Autodesk Inventor part; units mm, degrees
(part 2 of 3)
sketch "Sketch6" plane through (-41.727, 100.5291, 48.8096) normal (0.258819, 0.9659258, 0) x (0.9659258, -0.258819, 0)
  line L0 (0, 0) -> (0, 97.6191) projected
  line L1 (17.5553, 17.379) -> (17.5553, 16.4322)
  line L2 (17.5553, 16.4322) -> (12.0801, 13.6226)
  line L3 (12.0801, 13.6226) -> (17.5553, 13.6226)
  line L4 (17.5553, 13.6226) -> (17.5553, 12.8352)
  line L5 (17.5553, 12.8352) -> (11.2053, 12.8352)
  line L6 (11.2053, 12.8352) -> (11.2053, 14.0342)
  line L7 (11.2053, 14.0342) -> (16.2328, 16.5917)
  line L8 (16.2328, 16.5917) -> (11.2053, 16.5917)
  line L9 (11.2053, 16.5917) -> (11.2053, 17.379)
  line L10 (11.2053, 17.379) -> (17.5553, 17.379)
  line L11 (17.5553, 17.9811) -> (11.2053, 20.1218)
  line L12 (11.2053, 20.1218) -> (11.2053, 21.1612)
  line L13 (11.2053, 21.1612) -> (17.5553, 23.3019)
  line L14 (17.5553, 23.3019) -> (17.5553, 22.4117)
  line L15 (17.5553, 22.4117) -> (15.7799, 21.8354)
  line L16 (15.7799, 21.8354) -> (15.7799, 19.4117)
  line L17 (15.7799, 19.4117) -> (17.5553, 18.8353)
  line L18 (17.5553, 18.8353) -> (17.5553, 17.9811)
  line L19 (15.0595, 21.6038) -> (12.0698, 20.6209)
  line L20 (12.0698, 20.6209) -> (15.0595, 19.6432)
  line L21 (15.0595, 19.6432) -> (15.0595, 21.6038)
  spline S0 degree 2 poles (17.6685, 25.6742) (17.6685, 24.9846) (17.3803, 24.0172) (17.1745, 23.5901) knots 0 0 0 1 2 2 2
  line L22 (17.1745, 23.5901) -> (16.1144, 23.5901)
  line L23 (16.1144, 23.5901) -> (16.1144, 23.6518)
  spline S1 degree 2 poles (16.1144, 23.6518) (16.5055, 24.0687) (16.9378, 25.1236) (16.9378, 25.6124) knots 0 0 0 1 2 2 2
  spline S2 degree 2 poles (16.9378, 25.6124) (16.9378, 26.3123) (16.3563, 27.0275) (15.8777, 27.0275) knots 0 0 0 1 2 2 2
  spline S3 degree 2 poles (15.8777, 27.0275) (15.4969, 27.0275) (15.0235, 26.6519) (14.9051, 26.2454) knots 0 0 0 1 2 2 2
  spline S4 degree 2 poles (14.9051, 26.2454) (14.8228, 25.952) (14.7096, 25.4632) (14.617, 25.0978) knots 0 0 0 1 2 2 2
  spline S5 degree 2 poles (14.617, 25.0978) (14.5295, 24.7685) (14.2671, 24.2488) (14.0561, 24.0481) knots 0 0 0 1 2 2 2
  spline S6 degree 2 poles (14.0561, 24.0481) (13.8451, 23.8525) (13.2791, 23.6364) (12.9086, 23.6364) knots 0 0 0 1 2 2 2
  spline S7 degree 2 poles (12.9086, 23.6364) (12.1367, 23.6364) (11.0921, 24.8405) (11.0921, 25.7719) knots 0 0 0 1 2 2 2
  spline S8 degree 2 poles (11.0921, 25.7719) (11.0921, 26.3071) (11.303, 27.254) (11.5037, 27.6605) knots 0 0 0 1 2 2 2
  line L24 (11.5037, 27.6605) -> (12.5123, 27.6605)
  line L25 (12.5123, 27.6605) -> (12.5123, 27.5987)
  spline S9 degree 2 poles (12.5123, 27.5987) (12.2344, 27.2951) (11.8228, 26.3483) (11.8228, 25.8285) knots 0 0 0 1 2 2 2
  spline S10 degree 2 poles (11.8228, 25.8285) (11.8228, 25.2419) (12.3734, 24.5164) (12.8211, 24.5164) knots 0 0 0 1 2 2 2
  spline S11 degree 2 poles (12.8211, 24.5164) (13.2225, 24.5164) (13.701, 24.9435) (13.8091, 25.3448) knots 0 0 0 1 2 2 2
  spline S12 degree 2 poles (13.8091, 25.3448) (13.8811, 25.6124) (14.0664, 26.3894) (14.1436, 26.6467) knots 0 0 0 1 2 2 2
  spline S13 degree 2 poles (14.1436, 26.6467) (14.3442, 27.3003) (15.1522, 27.9075) (15.7439, 27.9075) knots 0 0 0 1 2 2 2
  spline S14 degree 2 poles (15.7439, 27.9075) (16.1196, 27.9075) (16.84, 27.6039) (17.0921, 27.3311) knots 0 0 0 1 2 2 2
  spline S15 degree 2 poles (17.0921, 27.3311) (17.37, 27.0275) (17.6685, 26.2557) (17.6685, 25.6742) knots 0 0 0 1 2 2 2
  line L26 (17.5553, 28.0824) -> (11.2053, 30.2231)
  line L27 (11.2053, 30.2231) -> (11.2053, 31.2626)
  line L28 (11.2053, 31.2626) -> (17.5553, 33.4033)
  line L29 (17.5553, 33.4033) -> (17.5553, 32.513)
  line L30 (17.5553, 32.513) -> (15.7799, 31.9367)
  line L31 (15.7799, 31.9367) -> (15.7799, 29.513)
  line L32 (15.7799, 29.513) -> (17.5553, 28.9367)
  line L33 (17.5553, 28.9367) -> (17.5553, 28.0824)
  line L34 (15.0595, 31.7051) -> (12.0698, 30.7223)
  line L35 (12.0698, 30.7223) -> (15.0595, 29.7446)
  line L36 (15.0595, 29.7446) -> (15.0595, 31.7051)
  spline S16 degree 2 poles (17.6685, 38.5028) (17.6685, 37.8133) (17.3803, 36.8458) (17.1745, 36.4187) knots 0 0 0 1 2 2 2
  line L37 (17.1745, 36.4187) -> (16.1144, 36.4187)
  line L38 (16.1144, 36.4187) -> (16.1144, 36.4805)
  spline S17 degree 2 poles (16.1144, 36.4805) (16.5055, 36.8973) (16.9378, 37.9522) (16.9378, 38.4411) knots 0 0 0 1 2 2 2
  spline S18 degree 2 poles (16.9378, 38.4411) (16.9378, 39.1409) (16.3563, 39.8562) (15.8777, 39.8562) knots 0 0 0 1 2 2 2
  spline S19 degree 2 poles (15.8777, 39.8562) (15.4969, 39.8562) (15.0235, 39.4805) (14.9051, 39.074) knots 0 0 0 1 2 2 2
  spline S20 degree 2 poles (14.9051, 39.074) (14.8228, 38.7807) (14.7096, 38.2918) (14.617, 37.9265) knots 0 0 0 1 2 2 2
  spline S21 degree 2 poles (14.617, 37.9265) (14.5295, 37.5971) (14.2671, 37.0774) (14.0561, 36.8767) knots 0 0 0 1 2 2 2
  spline S22 degree 2 poles (14.0561, 36.8767) (13.8451, 36.6812) (13.2791, 36.4651) (12.9086, 36.4651) knots 0 0 0 1 2 2 2
  spline S23 degree 2 poles (12.9086, 36.4651) (12.1367, 36.4651) (11.0921, 37.6692) (11.0921, 38.6006) knots 0 0 0 1 2 2 2
  spline S24 degree 2 poles (11.0921, 38.6006) (11.0921, 39.1358) (11.303, 40.0826) (11.5037, 40.4891) knots 0 0 0 1 2 2 2
  line L39 (11.5037, 40.4891) -> (12.5123, 40.4891)
  line L40 (12.5123, 40.4891) -> (12.5123, 40.4274)
  spline S25 degree 2 poles (12.5123, 40.4274) (12.2344, 40.1238) (11.8228, 39.1769) (11.8228, 38.6572) knots 0 0 0 1 2 2 2
  spline S26 degree 2 poles (11.8228, 38.6572) (11.8228, 38.0706) (12.3734, 37.345) (12.8211, 37.345) knots 0 0 0 1 2 2 2
  spline S27 degree 2 poles (12.8211, 37.345) (13.2225, 37.345) (13.701, 37.7721) (13.8091, 38.1735) knots 0 0 0 1 2 2 2
  spline S28 degree 2 poles (13.8091, 38.1735) (13.8811, 38.4411) (14.0664, 39.2181) (14.1436, 39.4754) knots 0 0 0 1 2 2 2
  spline S29 degree 2 poles (14.1436, 39.4754) (14.3442, 40.1289) (15.1522, 40.7361) (15.7439, 40.7361) knots 0 0 0 1 2 2 2
  spline S30 degree 2 poles (15.7439, 40.7361) (16.1196, 40.7361) (16.84, 40.4325) (17.0921, 40.1598) knots 0 0 0 1 2 2 2
  spline S31 degree 2 poles (17.0921, 40.1598) (17.37, 39.8562) (17.6685, 39.0843) (17.6685, 38.5028) knots 0 0 0 1 2 2 2
  line L41 (12.7902, 47.3074) -> (17.5553, 46.0981)
  line L42 (17.5553, 46.0981) -> (17.5553, 45.3571)
  line L43 (17.5553, 45.3571) -> (13.8811, 44.1941)
  line L44 (13.8811, 44.1941) -> (17.5553, 43.0363)
  line L45 (17.5553, 43.0363) -> (17.5553, 42.3005)
  line L46 (17.5553, 42.3005) -> (12.7902, 41.0809)
  line L47 (12.7902, 41.0809) -> (12.7902, 41.9145)
  line L48 (12.7902, 41.9145) -> (16.4798, 42.7585)
  line L49 (16.4798, 42.7585) -> (12.7902, 43.8854)
  line L50 (12.7902, 43.8854) -> (12.7902, 44.5492)
  line L51 (12.7902, 44.5492) -> (16.4798, 45.707)
  line L52 (16.4798, 45.707) -> (12.7902, 46.4995)
  line L53 (12.7902, 46.4995) -> (12.7902, 47.3074)
  spline S32 degree 2 poles (17.051, 50.6676) (17.123, 50.5699) (17.3803, 50.2405) (17.4575, 50.0862) knots 0 0 0 1 2 2 2
  spline S33 degree 2 poles (17.4575, 50.0862) (17.5707, 49.8752) (17.6891, 49.479) (17.6891, 49.1187) knots 0 0 0 1 2 2 2
  spline S34 degree 2 poles (17.6891, 49.1187) (17.6891, 48.8254) (17.4678, 48.2954) (17.2671, 48.0947) knots 0 0 0 1 2 2 2
  spline S35 degree 2 poles (17.2671, 48.0947) (17.0716, 47.9043) (16.4952, 47.6728) (16.1762, 47.6728) knots 0 0 0 1 2 2 2
  spline S36 degree 2 poles (16.1762, 47.6728) (15.6822, 47.6728) (14.9823, 48.0896) (14.7816, 48.5424) knots 0 0 0 1 2 2 2
  spline S37 degree 2 poles (14.7816, 48.5424) (14.5964, 48.9438) (14.4575, 50.0347) (14.4214, 50.6676) knots 0 0 0 1 2 2 2
  line L54 (14.4214, 50.6676) -> (14.2671, 50.6676)
  spline S38 degree 2 poles (14.2671, 50.6676) (13.9892, 50.6676) (13.6444, 50.4978) (13.5466, 50.3435) knots 0 0 0 1 2 2 2
  spline S39 degree 2 poles (13.5466, 50.3435) (13.4489, 50.1891) (13.3871, 49.7465) (13.3871, 49.5098) knots 0 0 0 1 2 2 2
  spline S40 degree 2 poles (13.3871, 49.5098) (13.3871, 49.232) (13.5518, 48.4807) (13.7113, 48.105) knots 0 0 0 1 2 2 2
  line L55 (13.7113, 48.105) -> (13.7113, 48.0587)
  line L56 (13.7113, 48.0587) -> (12.8931, 48.0587)
  spline S41 degree 2 poles (12.8931, 48.0587) (12.8314, 48.28) (12.677, 49.1085) (12.677, 49.515) knots 0 0 0 1 2 2 2
  spline S42 degree 2 poles (12.677, 49.515) (12.677, 50.009) (12.8314, 50.6831) (13.0321, 50.9507) knots 0 0 0 1 2 2 2
  spline S43 degree 2 poles (13.0321, 50.9507) (13.2276, 51.2131) (13.8502, 51.4704) (14.2979, 51.4704) knots 0 0 0 1 2 2 2
  line L57 (14.2979, 51.4704) -> (17.5553, 51.4704)
  line L58 (17.5553, 51.4704) -> (17.5553, 50.6676)
  line L59 (17.5553, 50.6676) -> (17.051, 50.6676)
  line L60 (16.382, 50.6676) -> (15.0595, 50.6676)
  spline S44 degree 2 poles (15.0595, 50.6676) (15.0853, 50.3795) (15.1727, 49.5098) (15.2551, 49.2371) knots 0 0 0 1 2 2 2
  spline S45 degree 2 poles (15.2551, 49.2371) (15.3528, 48.9181) (15.7594, 48.5012) (16.1196, 48.5012) knots 0 0 0 1 2 2 2
  spline S46 degree 2 poles (16.1196, 48.5012) (16.5312, 48.5012) (16.9481, 48.9644) (16.9481, 49.4069) knots 0 0 0 1 2 2 2
  spline S47 degree 2 poles (16.9481, 49.4069) (16.9481, 49.7826) (16.6239, 50.4001) (16.382, 50.6676) knots 0 0 0 1 2 2 2
  line L61 (13.6496, 55.124) -> (13.6496, 55.0828)
  spline S48 degree 2 poles (13.6496, 55.0828) (13.6238, 54.9902) (13.6135, 54.7895) (13.6135, 54.6505) knots 0 0 0 1 2 2 2
  spline S49 degree 2 poles (13.6135, 54.6505) (13.6135, 54.3264) (13.8966, 53.6883) (14.1744, 53.4001) knots 0 0 0 1 2 2 2
  line L62 (14.1744, 53.4001) -> (17.5553, 53.4001)
  line L63 (17.5553, 53.4001) -> (17.5553, 52.5973)
  line L64 (17.5553, 52.5973) -> (12.7902, 52.5973)
  line L65 (12.7902, 52.5973) -> (12.7902, 53.4001)
  line L66 (12.7902, 53.4001) -> (13.5003, 53.4001)
  spline S50 degree 2 poles (13.5003, 53.4001) (13.1092, 53.8375) (12.7902, 54.491) (12.7902, 54.7998) knots 0 0 0 1 2 2 2
  spline S51 degree 2 poles (12.7902, 54.7998) (12.7902, 54.9233) (12.8005, 55.0468) (12.8159, 55.124) knots 0 0 0 1 2 2 2
  line L67 (12.8159, 55.124) -> (13.6496, 55.124)
  line L68 (17.5553, 61.1498) -> (14.7971, 61.1498)
  spline S52 degree 2 poles (14.7971, 61.1498) (14.4678, 61.1498) (13.9069, 61.0983) (13.7525, 61.016) knots 0 0 0 1 2 2 2
  spline S53 degree 2 poles (13.7525, 61.016) (13.5827, 60.9337) (13.418, 60.6198) (13.418, 60.347) knots 0 0 0 1 2 2 2
  spline S54 degree 2 poles (13.418, 60.347) (13.418, 60.1) (13.7216, 59.534) (14.0098, 59.2355) knots 0 0 0 1 2 2 2
  spline S55 degree 2 poles (14.0098, 59.2355) (14.0818, 59.2407) (14.2825, 59.251) (14.4163, 59.251) knots 0 0 0 1 2 2 2
  line L69 (14.4163, 59.251) -> (17.5553, 59.251)
  line L70 (17.5553, 59.251) -> (17.5553, 58.4482)
  line L71 (17.5553, 58.4482) -> (14.7971, 58.4482)
  spline S56 degree 2 poles (14.7971, 58.4482) (14.4678, 58.4482) (13.9069, 58.3967) (13.7525, 58.3144) knots 0 0 0 1 2 2 2
  spline S57 degree 2 poles (13.7525, 58.3144) (13.5827, 58.2321) (13.418, 57.9182) (13.418, 57.6454) knots 0 0 0 1 2 2 2
  spline S58 degree 2 poles (13.418, 57.6454) (13.418, 57.3882) (13.7422, 56.817) (13.9943, 56.5494) knots 0 0 0 1 2 2 2
  line L72 (13.9943, 56.5494) -> (17.5553, 56.5494)
  line L73 (17.5553, 56.5494) -> (17.5553, 55.7466)
  line L74 (17.5553, 55.7466) -> (12.7902, 55.7466)
  line L75 (12.7902, 55.7466) -> (12.7902, 56.5494)
  line L76 (12.7902, 56.5494) -> (13.3151, 56.5494)
  spline S59 degree 2 poles (13.3151, 56.5494) (13.0012, 56.8633) (12.6564, 57.4808) (12.6564, 57.8513) knots 0 0 0 1 2 2 2
  spline S60 degree 2 poles (12.6564, 57.8513) (12.6564, 58.2732) (13.0423, 58.9268) (13.4797, 59.0966) knots 0 0 0 1 2 2 2
  spline S61 degree 2 poles (13.4797, 59.0966) (13.0732, 59.4619) (12.6564, 60.1515) (12.6564, 60.5529) knots 0 0 0 1 2 2 2
  spline S62 degree 2 poles (12.6564, 60.5529) (12.6564, 60.8616) (12.8468, 61.3659) (13.0629, 61.5512) knots 0 0 0 1 2 2 2
  spline S63 degree 2 poles (13.0629, 61.5512) (13.2791, 61.7416) (13.9274, 61.9525) (14.4163, 61.9525) knots 0 0 0 1 2 2 2
  line L77 (14.4163, 61.9525) -> (17.5553, 61.9525)
  line L78 (17.5553, 61.9525) -> (17.5553, 61.1498)
  spline S64 degree 2 poles (17.051, 65.7347) (17.123, 65.637) (17.3803, 65.3076) (17.4575, 65.1533) knots 0 0 0 1 2 2 2
  spline S65 degree 2 poles (17.4575, 65.1533) (17.5707, 64.9423) (17.6891, 64.5461) (17.6891, 64.1858) knots 0 0 0 1 2 2 2
  spline S66 degree 2 poles (17.6891, 64.1858) (17.6891, 63.8925) (17.4678, 63.3625) (17.2671, 63.1618) knots 0 0 0 1 2 2 2
  spline S67 degree 2 poles (17.2671, 63.1618) (17.0716, 62.9714) (16.4952, 62.7399) (16.1762, 62.7399) knots 0 0 0 1 2 2 2
  spline S68 degree 2 poles (16.1762, 62.7399) (15.6822, 62.7399) (14.9823, 63.1567) (14.7816, 63.6095) knots 0 0 0 1 2 2 2
  spline S69 degree 2 poles (14.7816, 63.6095) (14.5964, 64.0109) (14.4575, 65.1018) (14.4214, 65.7347) knots 0 0 0 1 2 2 2
  line L79 (14.4214, 65.7347) -> (14.2671, 65.7347)
  spline S70 degree 2 poles (14.2671, 65.7347) (13.9892, 65.7347) (13.6444, 65.5649) (13.5466, 65.4106) knots 0 0 0 1 2 2 2
  spline S71 degree 2 poles (13.5466, 65.4106) (13.4489, 65.2562) (13.3871, 64.8136) (13.3871, 64.5769) knots 0 0 0 1 2 2 2
  spline S72 degree 2 poles (13.3871, 64.5769) (13.3871, 64.299) (13.5518, 63.5478) (13.7113, 63.1721) knots 0 0 0 1 2 2 2
  line L80 (13.7113, 63.1721) -> (13.7113, 63.1258)
  line L81 (13.7113, 63.1258) -> (12.8931, 63.1258)
  spline S73 degree 2 poles (12.8931, 63.1258) (12.8314, 63.3471) (12.677, 64.1755) (12.677, 64.5821) knots 0 0 0 1 2 2 2
  spline S74 degree 2 poles (12.677, 64.5821) (12.677, 65.0761) (12.8314, 65.7502) (13.0321, 66.0178) knots 0 0 0 1 2 2 2
  spline S75 degree 2 poles (13.0321, 66.0178) (13.2276, 66.2802) (13.8502, 66.5375) (14.2979, 66.5375) knots 0 0 0 1 2 2 2
  line L82 (14.2979, 66.5375) -> (17.5553, 66.5375)
  line L83 (17.5553, 66.5375) -> (17.5553, 65.7347)
  line L84 (17.5553, 65.7347) -> (17.051, 65.7347)
  line L85 (16.382, 65.7347) -> (15.0595, 65.7347)
  spline S76 degree 2 poles (15.0595, 65.7347) (15.0853, 65.4466) (15.1727, 64.5769) (15.2551, 64.3042) knots 0 0 0 1 2 2 2
  spline S77 degree 2 poles (15.2551, 64.3042) (15.3528, 63.9852) (15.7594, 63.5683) (16.1196, 63.5683) knots 0 0 0 1 2 2 2
  spline S78 degree 2 poles (16.1196, 63.5683) (16.5312, 63.5683) (16.9481, 64.0315) (16.9481, 64.474) knots 0 0 0 1 2 2 2
  spline S79 degree 2 poles (16.9481, 64.474) (16.9481, 64.8497) (16.6239, 65.4672) (16.382, 65.7347) knots 0 0 0 1 2 2 2
  spline S80 degree 2 poles (17.6479, 69.1053) (17.6479, 68.4518) (16.9017, 67.7159) (16.0938, 67.7159) knots 0 0 0 1 2 2 2
  line L86 (16.0938, 67.7159) -> (13.454, 67.7159)
  line L87 (13.454, 67.7159) -> (13.454, 67.1756)
  line L88 (13.454, 67.1756) -> (12.7902, 67.1756)
  line L89 (12.7902, 67.1756) -> (12.7902, 67.7159)
  line L90 (12.7902, 67.7159) -> (11.4214, 67.7159)
  line L91 (11.4214, 67.7159) -> (11.4214, 68.5187)
  line L92 (11.4214, 68.5187) -> (12.7902, 68.5187)
  line L93 (12.7902, 68.5187) -> (12.7902, 69.9955)
  line L94 (12.7902, 69.9955) -> (13.454, 69.9955)
  line L95 (13.454, 69.9955) -> (13.454, 68.5187)
  line L96 (13.454, 68.5187) -> (15.7233, 68.5187)
  spline S81 degree 2 poles (15.7233, 68.5187) (16.0836, 68.5187) (16.4798, 68.5444) (16.6496, 68.6319) knots 0 0 0 1 2 2 2
  spline S82 degree 2 poles (16.6496, 68.6319) (16.7988, 68.7039) (16.9481, 69.0281) (16.9481, 69.306) knots 0 0 0 1 2 2 2
  spline S83 degree 2 poles (16.9481, 69.306) (16.9481, 69.5015) (16.8297, 69.8669) (16.7937, 69.9492) knots 0 0 0 1 2 2 2
  line L97 (16.7937, 69.9492) -> (16.7937, 69.9955)
  line L98 (16.7937, 69.9955) -> (17.5141, 69.9955)
  spline S84 degree 2 poles (17.5141, 69.9955) (17.5759, 69.7691) (17.6479, 69.306) (17.6479, 69.1053) knots 0 0 0 1 2 2 2
  line L99 (17.5553, 74.3283) -> (17.5553, 73.5256)
  line L100 (17.5553, 73.5256) -> (14.8383, 73.5256)
  spline S85 degree 2 poles (14.8383, 73.5256) (14.5089, 73.5256) (13.9429, 73.4638) (13.7731, 73.3712) knots 0 0 0 1 2 2 2
  spline S86 degree 2 poles (13.7731, 73.3712) (13.593, 73.2734) (13.418, 72.9235) (13.418, 72.6251) knots 0 0 0 1 2 2 2
  spline S87 degree 2 poles (13.418, 72.6251) (13.418, 72.3266) (13.737, 71.6937) (13.9943, 71.3901) knots 0 0 0 1 2 2 2
  line L101 (13.9943, 71.3901) -> (17.5553, 71.3901)
  line L102 (17.5553, 71.3901) -> (17.5553, 70.5873)
  line L103 (17.5553, 70.5873) -> (10.9222, 70.5873)
  line L104 (10.9222, 70.5873) -> (10.9222, 71.3901)
  line L105 (10.9222, 71.3901) -> (13.3202, 71.3901)
  spline S88 degree 2 poles (13.3202, 71.3901) (12.996, 71.7503) (12.6564, 72.445) (12.6564, 72.836) knots 0 0 0 1 2 2 2
  spline S89 degree 2 poles (12.6564, 72.836) (12.6564, 73.5359) (13.5827, 74.3283) (14.4626, 74.3283) knots 0 0 0 1 2 2 2
  line L106 (14.4626, 74.3283) -> (17.5553, 74.3283)
  spline S90 degree 2 poles (15.1727, 79.3713) (16.3769, 79.3713) (17.6891, 78.2135) (17.6891, 77.2461) knots 0 0 0 1 2 2 2
  spline S91 degree 2 poles (17.6891, 77.2461) (17.6891, 76.2529) (16.3357, 75.1157) (15.1727, 75.1157) knots 0 0 0 1 2 2 2
  spline S92 degree 2 poles (15.1727, 75.1157) (13.9789, 75.1157) (12.6564, 76.2889) (12.6564, 77.2461) knots 0 0 0 1 2 2 2
  spline S93 degree 2 poles (12.6564, 77.2461) (12.6564, 78.2135) (13.9737, 79.3713) (15.1727, 79.3713) knots 0 0 0 1 2 2 2
  spline S94 degree 2 poles (15.1727, 78.5428) (14.2465, 78.5428) (13.346, 77.8687) (13.346, 77.2461) knots 0 0 0 1 2 2 2
  spline S95 degree 2 poles (13.346, 77.2461) (13.346, 76.6234) (14.2465, 75.9441) (15.1727, 75.9441) knots 0 0 0 1 2 2 2
  spline S96 degree 2 poles (15.1727, 75.9441) (16.0733, 75.9441) (16.9995, 76.6234) (16.9995, 77.2461) knots 0 0 0 1 2 2 2
  spline S97 degree 2 poles (16.9995, 77.2461) (16.9995, 77.8636) (16.0887, 78.5428) (15.1727, 78.5428) knots 0 0 0 1 2 2 2
  line L107 (17.5553, 83.9357) -> (17.5553, 83.1329)
  line L108 (17.5553, 83.1329) -> (14.8383, 83.1329)
  spline S98 degree 2 poles (14.8383, 83.1329) (14.5089, 83.1329) (13.9429, 83.0712) (13.7731, 82.9785) knots 0 0 0 1 2 2 2
  spline S99 degree 2 poles (13.7731, 82.9785) (13.593, 82.8808) (13.418, 82.5309) (13.418, 82.2324) knots 0 0 0 1 2 2 2
  spline S100 degree 2 poles (13.418, 82.2324) (13.418, 81.9339) (13.737, 81.301) (13.9943, 80.9974) knots 0 0 0 1 2 2 2
  line L109 (13.9943, 80.9974) -> (17.5553, 80.9974)
  line L110 (17.5553, 80.9974) -> (17.5553, 80.1946)
  line L111 (17.5553, 80.1946) -> (12.7902, 80.1946)
  line L112 (12.7902, 80.1946) -> (12.7902, 80.9974)
  line L113 (12.7902, 80.9974) -> (13.3202, 80.9974)
  spline S101 degree 2 poles (13.3202, 80.9974) (12.996, 81.3576) (12.6564, 82.0523) (12.6564, 82.4434) knots 0 0 0 1 2 2 2
  spline S102 degree 2 poles (12.6564, 82.4434) (12.6564, 83.1432) (13.5827, 83.9357) (14.4626, 83.9357) knots 0 0 0 1 2 2 2
  line L114 (14.4626, 83.9357) -> (17.5553, 83.9357)
  point P0 (66.3241, 48.8096)
  point P1 (10.9222, 12.192)
  dimension "d33" = 12.192
  constraints: 1 other
  measures "d33" vertical distance of L0.start point (10.922, 12.192)
extrude "Extrusion6" add sketch "Sketch6" along normal blind 1.27
sketch "Sketch8" plane through (0, 0, 0) normal (0, -1, 0) x (1, 0, 0)
  arc A0 (-43.9323, 51.6673) -> (-45.7238, 48.8096) centre (-42.5488, 48.8096) ccw projected
  line L0 (-45.7238, -48.8096) -> (-45.7238, 48.8096) projected
  arc A1 (-45.7238, -48.8096) -> (-43.9323, -51.6673) centre (-42.5488, -48.8096) ccw projected
  line L1 (-2.3979, -71.7745) -> (-43.9323, -51.6673) projected
  arc A2 (-2.3979, -71.7745) -> (1.5596, -70.7755) centre (-1.0145, -68.9168) ccw projected
  line L2 (29.138, -32.5822) -> (1.5596, -70.7755) projected
  arc A3 (29.138, -32.5822) -> (29.7389, -30.7235) centre (26.5639, -30.7235) ccw projected
  line L3 (29.7389, 30.7235) -> (29.7389, -30.7235) projected
  arc A4 (29.7389, 30.7235) -> (29.138, 32.5822) centre (26.5639, 30.7235) ccw projected
  line L4 (1.5596, 70.7755) -> (29.138, 32.5822) projected
  arc A5 (1.5596, 70.7755) -> (-2.3979, 71.7745) centre (-1.0145, 68.9168) ccw projected
  line L5 (-43.9323, 51.6673) -> (-2.3979, 71.7745) projected
  line L6 (-28.5831, 49.7896) -> (-26.8927, 48.7793) projected
  line L7 (-28.5831, 51.8104) -> (-28.5831, 49.7896) projected
  line L8 (-26.8927, 52.8207) -> (-28.5831, 51.8104) projected
  line L9 (-25.2023, 51.8104) -> (-26.8927, 52.8207) projected
  line L10 (-25.2023, 49.7896) -> (-25.2023, 51.8104) projected
  line L11 (-26.8927, 48.7793) -> (-25.2023, 49.7896) projected
  line L12 (-28.1001, 24.6783) -> (-26.8927, 23.9566) projected
  line L13 (-28.1001, 26.1217) -> (-28.1001, 24.6783) projected
  line L14 (-26.8927, 26.8434) -> (-28.1001, 26.1217) projected
  line L15 (-25.6853, 26.1217) -> (-26.8927, 26.8434) projected
  line L16 (-25.6853, 24.6783) -> (-25.6853, 26.1217) projected
  line L17 (-26.8927, 23.9566) -> (-25.6853, 24.6783) projected
  line L18 (-27.8586, -0.5774) -> (-26.8927, -1.1547) projected
  line L19 (-27.8586, 0.5774) -> (-27.8586, -0.5774) projected
  line L20 (-26.8927, 1.1547) -> (-27.8586, 0.5774) projected
  line L21 (-25.9268, 0.5774) -> (-26.8927, 1.1547) projected
  line L22 (-25.9268, -0.5774) -> (-25.9268, 0.5774) projected
  line L23 (-26.8927, -1.1547) -> (-25.9268, -0.5774) projected
  line L24 (-28.0427, -26.0874) -> (-26.8927, -26.7748) projected
  line L25 (-28.0427, -24.7126) -> (-28.0427, -26.0874) projected
  line L26 (-26.8927, -24.0252) -> (-28.0427, -24.7126) projected
  line L27 (-25.7426, -24.7126) -> (-26.8927, -24.0252) projected
  line L28 (-25.7426, -26.0874) -> (-25.7426, -24.7126) projected
  line L29 (-26.8927, -26.7748) -> (-25.7426, -26.0874) projected
  line L30 (-26.126, -50.3417) -> (-26.8927, -49.8835) projected
  line L31 (-26.126, -51.2583) -> (-26.126, -50.3417) projected
  line L32 (-26.8927, -51.7165) -> (-26.126, -51.2583) projected
  line L33 (-27.6594, -51.2583) -> (-26.8927, -51.7165) projected
  line L34 (-27.6594, -50.3417) -> (-27.6594, -51.2583) projected
  line L35 (-26.8927, -49.8835) -> (-27.6594, -50.3417) projected
  line L36 (-8.861, 49.7896) -> (-7.1707, 48.7793) projected
  line L37 (-8.861, 51.8104) -> (-8.861, 49.7896) projected
  line L38 (-7.1707, 52.8207) -> (-8.861, 51.8104) projected
  line L39 (-21.6786, -56.7965) -> (5.3875, -56.7965)
  line L40 (5.3875, -56.7965) -> (-1.6231, -66.5056)
  line L41 (-1.6231, -66.5056) -> (-21.6786, -56.7965)
  line L42 (-2.3979, -71.7745) -> (-43.9323, -51.6673) projected
  line L43 (-19.3978, 57.9007) -> (4.5902, 57.9007)
  line L44 (4.5902, 57.9007) -> (-1.6231, 66.5056)
  line L45 (-1.6231, 66.5056) -> (-19.3978, 57.9007)
  line L46 (1.5596, 70.7755) -> (29.138, 32.5822) projected
  point P0 (0, 0)
  point P1 (-5.4803, 49.7896)
  point P2 (-5.4803, 51.8104)
  point P3 (-5.9633, 24.6783)
  point P4 (-5.9633, 26.1217)
  point P5 (-7.1707, 23.9566)
  point P6 (-7.1707, 26.8434)
  point P7 (-7.1707, -1.1547)
  point P8 (-7.1707, 1.1547)
  point P9 (-6.2047, 0.5774)
  point P10 (-6.2047, -0.5774)
  point P11 (-6.0206, -26.0874)
  point P12 (-6.0206, -24.7126)
  point P13 (-7.1707, -26.7748)
  point P14 (-7.1707, -24.0252)
  point P15 (-6.404, -51.2583)
  point P16 (-6.404, -50.3417)
  point P17 (-7.1707, -51.7165)
  point P18 (-7.1707, -49.8835)
  dimension "d38" = 5.08
  dimension "d39" = 5.08
  dimension "d40" = 5.08
  dimension "d41" = 5.08
  dimension "d42" = 5.08
  dimension "d43" = 5.08
  constraints: 12 end point, 4 parallel, 2 horizontal
  measures "d38" distance between parallel lines of L1 L41
  measures "d39" distance between parallel lines of L2 L40
  measures "d40" distance from line of L39 L32.start
  measures "d41" distance between parallel lines of L5 L45
  measures "d42" distance between parallel lines of L4 L44
  measures "d43" distance from line of L8.start L43
extrude "Extrusion8" cut sketch "Sketch8" against normal blind 76.2 contours L39 L40 L41 | L45 L44 L43
sketch "Sketch9" plane through (0, 0, 0) normal (0, -1, 0) x (1, 0, 0)
  line L0 (27.3857, 30.7235) -> (-0.1927, 68.9168) projected
  line L1 (27.3857, -30.7235) -> (27.3857, 30.7235) projected
  line L2 (-0.1927, -68.9168) -> (27.3857, -30.7235) projected
  line L3 (-41.727, -48.8096) -> (-0.1927, -68.9168) projected
  line L4 (-41.727, 48.8096) -> (-41.727, -48.8096) projected
  line L5 (-0.1927, 68.9168) -> (-41.727, 48.8096) projected
  line L6 (-8.861, 51.8104) -> (-8.861, 49.7896) projected
  line L7 (-8.861, 49.7896) -> (-7.1707, 48.7793) projected
  line L8 (-7.1707, 48.7793) -> (-5.4803, 49.7896) projected
  line L9 (-5.4803, 49.7896) -> (-5.4803, 51.8104) projected
  line L10 (-5.4803, 51.8104) -> (-7.1707, 52.8207) projected
  line L11 (-7.1707, 52.8207) -> (-8.861, 51.8104) projected
  line L12 (-6.404, -51.2583) -> (-6.404, -50.3417) projected
  line L13 (-6.404, -50.3417) -> (-7.1707, -49.8835) projected
  line L14 (-7.1707, -49.8835) -> (-7.9374, -50.3417) projected
  line L15 (-7.9374, -50.3417) -> (-7.9374, -51.2583) projected
  line L16 (-7.9374, -51.2583) -> (-7.1707, -51.7165) projected
  line L17 (-7.1707, -51.7165) -> (-6.404, -51.2583) projected
  line L18 (-8.3207, -24.7126) -> (-8.3207, -26.0874) projected
  line L19 (-8.3207, -26.0874) -> (-7.1707, -26.7748) projected
  line L20 (-7.1707, -26.7748) -> (-6.0206, -26.0874) projected
  line L21 (-6.0206, -26.0874) -> (-6.0206, -24.7126) projected
  line L22 (-6.0206, -24.7126) -> (-7.1707, -24.0252) projected
  line L23 (-7.1707, -24.0252) -> (-8.3207, -24.7126) projected
  line L24 (-8.1366, 0.5774) -> (-8.1366, -0.5774) projected
  line L25 (-8.1366, -0.5774) -> (-7.1707, -1.1547) projected
  line L26 (-7.1707, -1.1547) -> (-6.2047, -0.5774) projected
  line L27 (-6.2047, -0.5774) -> (-6.2047, 0.5774) projected
  line L28 (-6.2047, 0.5774) -> (-7.1707, 1.1547) projected
  line L29 (-7.1707, 1.1547) -> (-8.1366, 0.5774) projected
  line L30 (-8.3781, 26.1217) -> (-8.3781, 24.6783) projected
  line L31 (-8.3781, 24.6783) -> (-7.1707, 23.9566) projected
  line L32 (-7.1707, 23.9566) -> (-5.9633, 24.6783) projected
  line L33 (-5.9633, 24.6783) -> (-5.9633, 26.1217) projected
  line L34 (-5.9633, 26.1217) -> (-7.1707, 26.8434) projected
  line L35 (-7.1707, 26.8434) -> (-8.3781, 26.1217) projected
  line L36 (-15.0762, -56.7615) -> (-15.0762, -56.4923) projected
  line L37 (-15.0762, -56.4923) -> (-16.2214, -56.4034) projected
  line L38 (-16.2214, -56.4034) -> (-16.2214, -56.8504) projected
  line L39 (-16.2214, -56.8504) -> (-15.0762, -56.7615) projected
  line L40 (-13.146, -51.288) -> (-13.4467, -51.288) projected
  line L41 (-13.4467, -51.288) -> (-13.4467, -51.8412) projected
  line L42 (-13.4467, -51.8412) -> (-15.4198, -51.8412) projected
  line L43 (-15.4198, -51.8412) -> (-15.4198, -51.288) projected
  line L44 (-15.4198, -51.288) -> (-15.6894, -51.288) projected
  line L45 (-16.0997, -51.9178) -> (-16.0997, -52.234) projected
  line L46 (-16.0997, -52.234) -> (-13.4467, -52.234) projected
  line L47 (-13.4467, -52.234) -> (-13.4467, -52.7749) projected
  line L48 (-13.4467, -52.7749) -> (-13.146, -52.7749) projected
  line L49 (-13.146, -52.7749) -> (-13.146, -51.288) projected
  line L50 (-13.146, -47.3977) -> (-13.4467, -47.3977) projected
  line L51 (-13.4467, -47.3977) -> (-13.4467, -47.951) projected
  line L52 (-13.4467, -47.951) -> (-15.4198, -47.951) projected
  line L53 (-15.4198, -47.951) -> (-15.4198, -47.3977) projected
  line L54 (-15.4198, -47.3977) -> (-15.6894, -47.3977) projected
  line L55 (-16.0997, -48.0275) -> (-16.0997, -48.3437) projected
  line L56 (-16.0997, -48.3437) -> (-13.4467, -48.3437) projected
  line L57 (-13.4467, -48.3437) -> (-13.4467, -48.8846) projected
  line L58 (-13.4467, -48.8846) -> (-13.146, -48.8846) projected
  line L59 (-13.146, -48.8846) -> (-13.146, -47.3977) projected
  line L60 (-15.0762, -31.0544) -> (-15.0762, -30.7852) projected
  line L61 (-15.0762, -30.7852) -> (-16.2214, -30.6962) projected
  line L62 (-16.2214, -30.6962) -> (-16.2214, -31.1433) projected
  line L63 (-16.2214, -31.1433) -> (-15.0762, -31.0544) projected
  line L64 (-15.5534, -25.4252) -> (-15.5534, -25.4005) projected
  line L65 (-15.5534, -25.4005) -> (-15.9709, -25.4005) projected
  line L66 (-14.7827, -26.5466) -> (-14.7541, -26.5466) projected
  line L67 (-13.2653, -25.3165) -> (-13.6829, -25.3165) projected
  line L68 (-13.6829, -25.3165) -> (-13.6829, -25.3462) projected
  line L69 (-14.5799, -26.1119) -> (-14.5799, -25.939) projected
  line L70 (-14.5799, -25.939) -> (-14.9068, -25.939) projected
  line L71 (-14.9068, -25.939) -> (-14.9068, -26.0748) projected
  line L72 (-15.5534, -21.5349) -> (-15.5534, -21.5102) projected
  line L73 (-15.5534, -21.5102) -> (-15.9709, -21.5102) projected
  line L74 (-14.7827, -22.6563) -> (-14.7541, -22.6563) projected
  line L75 (-13.2653, -21.4263) -> (-13.6829, -21.4263) projected
  line L76 (-13.6829, -21.4263) -> (-13.6829, -21.4559) projected
  line L77 (-14.5799, -22.2216) -> (-14.5799, -22.0487) projected
  line L78 (-14.5799, -22.0487) -> (-14.9068, -22.0487) projected
  line L79 (-14.9068, -22.0487) -> (-14.9068, -22.1846) projected
  line L80 (-14.6706, -2.6536) -> (-13.2152, -2.6536) projected
  line L81 (-13.2152, -2.6536) -> (-13.2152, -2.2683) projected
  line L82 (-13.2152, -2.2683) -> (-14.494, -2.2683) projected
  line L83 (-14.8662, -1.3568) -> (-13.2152, -1.3568) projected
  line L84 (-13.2152, -1.3568) -> (-13.2152, -0.9715) projected
  line L85 (-13.2152, -0.9715) -> (-15.4245, -0.9715) projected
  line L86 (-15.4245, -0.9715) -> (-15.4245, -1.3568) projected
  line L87 (-15.4245, -1.3568) -> (-15.1812, -1.3568) projected
  line L88 (-14.6706, -3.9504) -> (-13.2152, -3.9504) projected
  line L89 (-13.2152, -3.9504) -> (-13.2152, -3.565) projected
  line L90 (-13.2152, -3.565) -> (-14.494, -3.565) projected
  line L91 (-13.2152, 6.2385) -> (-13.6327, 6.2385) projected
  line L92 (-15.6249, 6.152) -> (-15.6249, 6.1742) projected
  line L93 (-15.6249, 6.1742) -> (-16.0448, 6.1742) projected
  line L94 (-13.5564, 5.8556) -> (-13.5564, 4.3588) projected
  line L95 (-13.5564, 4.3588) -> (-13.2152, 4.3588) projected
  line L96 (-13.2152, 4.3588) -> (-13.2152, 6.2385) projected
  line L97 (-14.6706, 22.6526) -> (-13.2152, 22.6526) projected
  line L98 (-13.2152, 22.6526) -> (-13.2152, 23.0379) projected
  line L99 (-13.2152, 23.0379) -> (-14.494, 23.0379) projected
  line L100 (-14.8662, 23.9494) -> (-13.2152, 23.9494) projected
  line L101 (-13.2152, 23.9494) -> (-13.2152, 24.3347) projected
  line L102 (-13.2152, 24.3347) -> (-15.4245, 24.3347) projected
  line L103 (-15.4245, 24.3347) -> (-15.4245, 23.9494) projected
  line L104 (-15.4245, 23.9494) -> (-15.1812, 23.9494) projected
  line L105 (-14.6706, 21.3559) -> (-13.2152, 21.3559) projected
  line L106 (-13.2152, 21.3559) -> (-13.2152, 21.7412) projected
  line L107 (-13.2152, 21.7412) -> (-14.494, 21.7412) projected
  line L108 (-13.2152, 29.092) -> (-13.7783, 29.092) projected
  line L109 (-13.7783, 29.092) -> (-13.7783, 28.6029) projected
  line L110 (-13.7783, 28.6029) -> (-13.2152, 28.6029) projected
  line L111 (-13.2152, 28.6029) -> (-13.2152, 29.092) projected
  line L112 (-14.6706, 44.5211) -> (-13.2152, 44.5211) projected
  line L113 (-13.2152, 44.5211) -> (-13.2152, 44.9064) projected
  line L114 (-13.2152, 44.9064) -> (-14.494, 44.9064) projected
  line L115 (-14.8662, 45.8179) -> (-13.2152, 45.8179) projected
  line L116 (-13.2152, 45.8179) -> (-13.2152, 46.2032) projected
  line L117 (-13.2152, 46.2032) -> (-15.4245, 46.2032) projected
  line L118 (-15.4245, 46.2032) -> (-15.4245, 45.8179) projected
  line L119 (-15.4245, 45.8179) -> (-15.1812, 45.8179) projected
  line L120 (-14.6706, 43.2244) -> (-13.2152, 43.2244) projected
  line L121 (-13.2152, 43.2244) -> (-13.2152, 43.6097) projected
  line L122 (-13.2152, 43.6097) -> (-14.494, 43.6097) projected
  line L123 (-13.3202, 53.344) -> (-13.7377, 53.344) projected
  line L124 (-13.7377, 53.344) -> (-13.7377, 53.3144) projected
  line L125 (-14.642, 53.2181) -> (-16.1594, 53.2181) projected
  line L126 (-16.1594, 53.2181) -> (-16.1594, 51.5459) projected
  line L127 (-16.1594, 51.5459) -> (-15.8134, 51.5459) projected
  line L128 (-15.8134, 51.5459) -> (-15.8134, 52.8253) projected
  line L129 (-15.8134, 52.8253) -> (-15.0285, 52.8253) projected
  line L130 (-15.6225, 56.849) -> (-15.6225, 56.8737) projected
  line L131 (-15.6225, 56.8737) -> (-16.0401, 56.8737) projected
  line L132 (-14.8519, 55.7276) -> (-14.8233, 55.7276) projected
  line L133 (-13.3345, 56.9577) -> (-13.752, 56.9577) projected
  line L134 (-13.752, 56.9577) -> (-13.752, 56.928) projected
  line L135 (-14.6491, 56.1623) -> (-14.6491, 56.3352) projected
  line L136 (-14.6491, 56.3352) -> (-14.976, 56.3352) projected
  line L137 (-14.976, 56.3352) -> (-14.976, 56.1994) projected
  line L138 (-13.2152, 54.4802) -> (-13.7783, 54.4802) projected
  line L139 (-13.7783, 54.4802) -> (-13.7783, 53.9912) projected
  line L140 (-13.7783, 53.9912) -> (-13.2152, 53.9912) projected
  line L141 (-13.2152, 53.9912) -> (-13.2152, 54.4802) projected
  line L142 (-14.6706, 48.0409) -> (-13.2152, 48.0409) projected
  line L143 (-13.2152, 48.0409) -> (-13.2152, 48.4262) projected
  line L144 (-13.2152, 48.4262) -> (-14.494, 48.4262) projected
  line L145 (-14.8662, 49.3377) -> (-13.2152, 49.3377) projected
  line L146 (-13.2152, 49.3377) -> (-13.2152, 49.723) projected
  line L147 (-13.2152, 49.723) -> (-15.4245, 49.723) projected
  line L148 (-15.4245, 49.723) -> (-15.4245, 49.3377) projected
  line L149 (-15.4245, 49.3377) -> (-15.1812, 49.3377) projected
  line L150 (-14.6706, 46.7441) -> (-13.2152, 46.7441) projected
  line L151 (-13.2152, 46.7441) -> (-13.2152, 47.1295) projected
  line L152 (-13.2152, 47.1295) -> (-14.494, 47.1295) projected
  line L153 (-13.2152, 31.5447) -> (-13.6327, 31.5447) projected
  line L154 (-15.6249, 31.4582) -> (-15.6249, 31.4805) projected
  line L155 (-15.6249, 31.4805) -> (-16.0448, 31.4805) projected
  line L156 (-13.5564, 31.1618) -> (-13.5564, 29.665) projected
  line L157 (-13.5564, 29.665) -> (-13.2152, 29.665) projected
  line L158 (-13.2152, 29.665) -> (-13.2152, 31.5447) projected
  line L159 (-13.3202, 27.9557) -> (-13.7377, 27.9557) projected
  line L160 (-13.7377, 27.9557) -> (-13.7377, 27.9261) projected
  line L161 (-14.642, 27.8298) -> (-16.1594, 27.8298) projected
  line L162 (-16.1594, 27.8298) -> (-16.1594, 26.1576) projected
  line L163 (-16.1594, 26.1576) -> (-15.8134, 26.1576) projected
  line L164 (-15.8134, 26.1576) -> (-15.8134, 27.437) projected
  line L165 (-15.8134, 27.437) -> (-15.0285, 27.437) projected
  line L166 (-14.6706, 19.1328) -> (-13.2152, 19.1328) projected
  line L167 (-13.2152, 19.1328) -> (-13.2152, 19.5182) projected
  line L168 (-13.2152, 19.5182) -> (-14.494, 19.5182) projected
  line L169 (-14.8662, 20.4296) -> (-13.2152, 20.4296) projected
  line L170 (-13.2152, 20.4296) -> (-13.2152, 20.8149) projected
  line L171 (-13.2152, 20.8149) -> (-15.4245, 20.8149) projected
  line L172 (-15.4245, 20.8149) -> (-15.4245, 20.4296) projected
  line L173 (-15.4245, 20.4296) -> (-15.1812, 20.4296) projected
  line L174 (-14.6706, 17.8361) -> (-13.2152, 17.8361) projected
  line L175 (-13.2152, 17.8361) -> (-13.2152, 18.2214) projected
  line L176 (-13.2152, 18.2214) -> (-14.494, 18.2214) projected
  line L177 (-13.2152, 3.7857) -> (-13.7783, 3.7857) projected
  line L178 (-13.7783, 3.7857) -> (-13.7783, 3.2967) projected
  line L179 (-13.7783, 3.2967) -> (-13.2152, 3.2967) projected
  line L180 (-13.2152, 3.2967) -> (-13.2152, 3.7857) projected
  line L181 (-14.6706, -6.1734) -> (-13.2152, -6.1734) projected
  line L182 (-13.2152, -6.1734) -> (-13.2152, -5.7881) projected
  line L183 (-13.2152, -5.7881) -> (-14.494, -5.7881) projected
  line L184 (-14.8662, -4.8766) -> (-13.2152, -4.8766) projected
  line L185 (-13.2152, -4.8766) -> (-13.2152, -4.4913) projected
  line L186 (-13.2152, -4.4913) -> (-15.4245, -4.4913) projected
  line L187 (-15.4245, -4.4913) -> (-15.4245, -4.8766) projected
  line L188 (-15.4245, -4.8766) -> (-15.1812, -4.8766) projected
  line L189 (-14.6706, -7.4701) -> (-13.2152, -7.4701) projected
  line L190 (-13.2152, -7.4701) -> (-13.2152, -7.0848) projected
  line L191 (-13.2152, -7.0848) -> (-14.494, -7.0848) projected
  line L192 (-12.5066, -23.8123) -> (-12.5066, -23.4665) projected
  line L193 (-12.5066, -23.4665) -> (-16.2214, -24.6546) projected
  line L194 (-16.2214, -24.6546) -> (-16.2214, -25.0053) projected
  line L195 (-16.2214, -25.0053) -> (-12.5066, -23.8123) projected
  line L196 (-13.146, -27.6285) -> (-13.5636, -27.6285) projected
  line L197 (-15.5557, -27.7149) -> (-15.5557, -27.6927) projected
  line L198 (-15.5557, -27.6927) -> (-15.9757, -27.6927) projected
  line L199 (-13.4872, -28.0113) -> (-13.4872, -29.5082) projected
  line L200 (-13.4872, -29.5082) -> (-13.146, -29.5082) projected
  line L201 (-13.146, -29.5082) -> (-13.146, -27.6285) projected
  line L202 (-15.0762, -30.2837) -> (-15.0762, -30.0145) projected
  line L203 (-15.0762, -30.0145) -> (-16.2214, -29.9256) projected
  line L204 (-16.2214, -29.9256) -> (-16.2214, -30.3727) projected
  line L205 (-16.2214, -30.3727) -> (-15.0762, -30.2837) projected
  line L206 (-12.5066, -49.5194) -> (-12.5066, -49.1736) projected
  line L207 (-12.5066, -49.1736) -> (-16.2214, -50.3617) projected
  line L208 (-16.2214, -50.3617) -> (-16.2214, -50.7125) projected
  line L209 (-16.2214, -50.7125) -> (-12.5066, -49.5194) projected
  line L210 (-16.1045, -54.9979) -> (-15.7251, -54.9979) projected
  line L211 (-15.7251, -54.9979) -> (-15.7251, -54.9806) projected
  line L212 (-15.0762, -55.9909) -> (-15.0762, -55.7216) projected
  line L213 (-15.0762, -55.7216) -> (-16.2214, -55.6327) projected
  line L214 (-16.2214, -55.6327) -> (-16.2214, -56.0798) projected
  line L215 (-16.2214, -56.0798) -> (-15.0762, -55.9909) projected
  line L216 (-24.77, -34.3234) -> (-27.3944, -34.3234) projected
  line L217 (-28.2096, -32.1878) -> (-24.77, -32.1878) projected
  line L218 (-24.77, -32.1878) -> (-24.77, -31.3851) projected
  line L219 (-24.77, -31.3851) -> (-29.3727, -31.3851) projected
  line L220 (-29.3727, -31.3851) -> (-29.3727, -32.1878) projected
  line L221 (-29.3727, -32.1878) -> (-28.8607, -32.1878) projected
  line L222 (-27.7572, -35.1261) -> (-24.77, -35.1261) projected
  line L223 (-24.77, -35.1261) -> (-24.77, -34.3234) projected
  line L224 (-26.1816, -18.9063) -> (-28.7315, -18.9063) projected
  line L225 (-28.7315, -18.9063) -> (-28.7315, -18.366) projected
  line L226 (-28.7315, -18.366) -> (-29.3727, -18.366) projected
  line L227 (-29.3727, -18.366) -> (-29.3727, -18.9063) projected
  line L228 (-29.3727, -18.9063) -> (-30.6948, -18.9063) projected
  line L229 (-30.6948, -18.9063) -> (-30.6948, -19.7091) projected
  line L230 (-30.6948, -19.7091) -> (-29.3727, -19.7091) projected
  line L231 (-29.3727, -19.7091) -> (-29.3727, -21.186) projected
  line L232 (-29.3727, -21.186) -> (-28.7315, -21.186) projected
  line L233 (-28.7315, -21.186) -> (-28.7315, -19.7091) projected
  line L234 (-28.7315, -19.7091) -> (-26.5395, -19.7091) projected
  line L235 (-25.5056, -21.1396) -> (-25.5056, -21.186) projected
  line L236 (-25.5056, -21.186) -> (-24.8097, -21.186) projected
  line L237 (-27.797, -16.9252) -> (-27.9461, -16.9252) projected
  line L238 (-28.4829, -14.3625) -> (-28.4829, -14.3162) projected
  line L239 (-28.4829, -14.3162) -> (-29.2732, -14.3162) projected
  line L240 (-27.9163, -17.7279) -> (-24.77, -17.7279) projected
  line L241 (-24.77, -17.7279) -> (-24.77, -16.9252) projected
  line L242 (-24.77, -16.9252) -> (-25.2571, -16.9252) projected
  line L243 (-28.0356, -4.5905) -> (-24.77, -4.5905) projected
  line L244 (-24.77, -4.5905) -> (-24.77, -3.7878) projected
  line L245 (-24.77, -3.7878) -> (-29.3727, -3.7878) projected
  line L246 (-29.3727, -3.7878) -> (-29.3727, -4.5905) projected
  line L247 (-29.3727, -4.5905) -> (-28.6867, -4.5905) projected
  line L248 (-29.3478, -6.3144) -> (-28.5426, -6.3144) projected
  line L249 (-28.5426, -6.3144) -> (-28.5426, -6.2732) projected
  line L250 (-27.797, -1.8581) -> (-27.9461, -1.8581) projected
  line L251 (-28.4829, 0.7046) -> (-28.4829, 0.7509) projected
  line L252 (-28.4829, 0.7509) -> (-29.2732, 0.7509) projected
  line L253 (-27.9163, -2.6608) -> (-24.77, -2.6608) projected
  line L254 (-24.77, -2.6608) -> (-24.77, -1.8581) projected
  line L255 (-24.77, -1.8581) -> (-25.2571, -1.8581) projected
  line L256 (-25.1378, 12.3908) -> (-26.1617, 12.3908) projected
  line L257 (-26.1617, 12.3908) -> (-26.1617, 12.3291) projected
  line L258 (-30.6153, 8.3204) -> (-29.6411, 8.3204) projected
  line L259 (-29.6411, 8.3204) -> (-29.6411, 8.3822) projected
  line L260 (-30.9036, 18.5864) -> (-30.9036, 17.547) projected
  line L261 (-30.9036, 17.547) -> (-24.77, 15.4063) projected
  line L262 (-24.77, 15.4063) -> (-24.77, 16.2965) projected
  line L263 (-24.77, 16.2965) -> (-26.4848, 16.8729) projected
  line L264 (-26.4848, 16.8729) -> (-26.4848, 19.2966) projected
  line L265 (-26.4848, 19.2966) -> (-24.77, 19.8729) projected
  line L266 (-24.77, 19.8729) -> (-24.77, 20.7271) projected
  line L267 (-24.77, 20.7271) -> (-30.9036, 18.5864) projected
  line L268 (-24.77, 32.3774) -> (-30.0586, 35.187) projected
  line L269 (-30.0586, 35.187) -> (-24.77, 35.187) projected
  line L270 (-24.77, 35.187) -> (-24.77, 35.9743) projected
  line L271 (-24.77, 35.9743) -> (-30.9036, 35.9743) projected
  line L272 (-30.9036, 35.9743) -> (-30.9036, 34.7753) projected
  line L273 (-30.9036, 34.7753) -> (-26.0474, 32.2178) projected
  line L274 (-26.0474, 32.2178) -> (-30.9036, 32.2178) projected
  line L275 (-30.9036, 32.2178) -> (-30.9036, 31.4305) projected
  line L276 (-30.9036, 31.4305) -> (-24.77, 31.4305) projected
  line L277 (-24.77, 31.4305) -> (-24.77, 32.3774) projected
  line L278 (-30.9036, 28.6878) -> (-30.9036, 27.6483) projected
  line L279 (-30.9036, 27.6483) -> (-24.77, 25.5076) projected
  line L280 (-24.77, 25.5076) -> (-24.77, 26.3979) projected
  line L281 (-24.77, 26.3979) -> (-26.4848, 26.9742) projected
  line L282 (-26.4848, 26.9742) -> (-26.4848, 29.3979) projected
  line L283 (-26.4848, 29.3979) -> (-24.77, 29.9743) projected
  line L284 (-24.77, 29.9743) -> (-24.77, 30.8285) projected
  line L285 (-24.77, 30.8285) -> (-30.9036, 28.6878) projected
  line L286 (-25.1378, 25.2195) -> (-26.1617, 25.2195) projected
  line L287 (-26.1617, 25.2195) -> (-26.1617, 25.1577) projected
  line L288 (-30.6153, 21.1491) -> (-29.6411, 21.1491) projected
  line L289 (-29.6411, 21.1491) -> (-29.6411, 21.2108) projected
  line L290 (-24.77, 2.7114) -> (-24.77, 3.4525) projected
  line L291 (-24.77, 3.4525) -> (-28.3189, 4.6154) projected
  line L292 (-28.3189, 4.6154) -> (-24.77, 5.7732) projected
  line L293 (-24.77, 5.7732) -> (-24.77, 6.5091) projected
  line L294 (-24.77, 6.5091) -> (-29.3727, 7.7287) projected
  line L295 (-29.3727, 7.7287) -> (-29.3727, 6.895) projected
  line L296 (-29.3727, 6.895) -> (-25.8088, 6.0511) projected
  line L297 (-25.8088, 6.0511) -> (-29.3727, 4.9242) projected
  line L298 (-29.3727, 4.9242) -> (-29.3727, 4.2604) projected
  line L299 (-29.3727, 4.2604) -> (-25.8088, 3.1025) projected
  line L300 (-25.8088, 3.1025) -> (-29.3727, 2.3101) projected
  line L301 (-29.3727, 2.3101) -> (-29.3727, 1.5022) projected
  line L302 (-29.3727, 1.5022) -> (-24.77, 2.7114) projected
  line L303 (-27.802, -10.4414) -> (-24.77, -10.4414) projected
  line L304 (-24.77, -10.4414) -> (-24.77, -9.6386) projected
  line L305 (-24.77, -9.6386) -> (-27.4342, -9.6386) projected
  line L306 (-28.2096, -7.7398) -> (-24.77, -7.7398) projected
  line L307 (-24.77, -7.7398) -> (-24.77, -6.9371) projected
  line L308 (-24.77, -6.9371) -> (-29.3727, -6.9371) projected
  line L309 (-29.3727, -6.9371) -> (-29.3727, -7.7398) projected
  line L310 (-29.3727, -7.7398) -> (-28.8657, -7.7398) projected
  line L311 (-27.802, -13.143) -> (-24.77, -13.143) projected
  line L312 (-24.77, -13.143) -> (-24.77, -12.3402) projected
  line L313 (-24.77, -12.3402) -> (-27.4342, -12.3402) projected
  line L314 (-24.77, -24.716) -> (-27.3944, -24.716) projected
  line L315 (-28.2096, -22.5805) -> (-24.77, -22.5805) projected
  line L316 (-24.77, -22.5805) -> (-24.77, -21.7777) projected
  line L317 (-24.77, -21.7777) -> (-31.177, -21.7777) projected
  line L318 (-31.177, -21.7777) -> (-31.177, -22.5805) projected
  line L319 (-31.177, -22.5805) -> (-28.8607, -22.5805) projected
  line L320 (-27.7572, -25.5188) -> (-24.77, -25.5188) projected
  line L321 (-24.77, -25.5188) -> (-24.77, -24.716) projected
  line L322 (-28.5831, 49.7896) -> (-26.8927, 48.7793) projected
  line L323 (-28.5831, 51.8104) -> (-28.5831, 49.7896) projected
  line L324 (-26.8927, 52.8207) -> (-28.5831, 51.8104) projected
  line L325 (-25.2023, 51.8104) -> (-26.8927, 52.8207) projected
  line L326 (-25.2023, 49.7896) -> (-25.2023, 51.8104) projected
  line L327 (-26.8927, 48.7793) -> (-25.2023, 49.7896) projected
  line L328 (-28.1001, 24.6783) -> (-26.8927, 23.9566) projected
  line L329 (-28.1001, 26.1217) -> (-28.1001, 24.6783) projected
  line L330 (-26.8927, 26.8434) -> (-28.1001, 26.1217) projected
  line L331 (-25.6853, 26.1217) -> (-26.8927, 26.8434) projected
  line L332 (-25.6853, 24.6783) -> (-25.6853, 26.1217) projected
  line L333 (-26.8927, 23.9566) -> (-25.6853, 24.6783) projected
  line L334 (-27.8586, -0.5774) -> (-26.8927, -1.1547) projected
  line L335 (-27.8586, 0.5774) -> (-27.8586, -0.5774) projected
  line L336 (-26.8927, 1.1547) -> (-27.8586, 0.5774) projected
  line L337 (-25.9268, 0.5774) -> (-26.8927, 1.1547) projected
  line L338 (-25.9268, -0.5774) -> (-25.9268, 0.5774) projected
  line L339 (-26.8927, -1.1547) -> (-25.9268, -0.5774) projected
  line L340 (-28.0427, -26.0874) -> (-26.8927, -26.7748) projected
  line L341 (-28.0427, -24.7126) -> (-28.0427, -26.0874) projected
  line L342 (-26.8927, -24.0252) -> (-28.0427, -24.7126) projected
  line L343 (-25.7426, -24.7126) -> (-26.8927, -24.0252) projected
  line L344 (-25.7426, -26.0874) -> (-25.7426, -24.7126) projected
  line L345 (-26.8927, -26.7748) -> (-25.7426, -26.0874) projected
  line L346 (-26.126, -50.3417) -> (-26.8927, -49.8835) projected
  line L347 (-26.126, -51.2583) -> (-26.126, -50.3417) projected
  line L348 (-26.8927, -51.7165) -> (-26.126, -51.2583) projected
  line L349 (-27.6594, -51.2583) -> (-26.8927, -51.7165) projected
  line L350 (-27.6594, -50.3417) -> (-27.6594, -51.2583) projected
  line L351 (-26.8927, -49.8835) -> (-27.6594, -50.3417) projected
  line L352 (-21.6786, -56.7965) -> (5.3875, -56.7965) projected
  line L353 (5.3875, -56.7965) -> (24.6589, -30.1076)
  line L354 (24.6589, -30.1076) -> (24.6589, 30.1076)
  line L355 (4.5902, 57.9007) -> (-19.3978, 57.9007) projected
  line L356 (24.6589, 30.1076) -> (4.5902, 57.9007)
  line L357 (4.5902, 57.9007) -> (-0.4003, 57.9007)
  line L358 (-0.4003, 57.9007) -> (-0.4003, -56.7965)
  line L359 (5.3875, -56.7965) -> (-1.6231, -66.5056) projected
  line L360 (-0.4003, -56.7965) -> (5.3875, -56.7965)
  line L361 (29.7389, 30.7235) -> (29.7389, -30.7235) projected
  point P0 (0, 0)
  dimension "d46" = 5.08
  dimension "d49" = 5.08
  constraints: 12 end point, 3 parallel, 2 point on line, 1 horizontal, 1 perpendicular, 297 other
  measures "d46" distance between parallel lines of L9 L358
  measures "d49" distance between parallel lines of L361 L354
extrude "Extrusion9" cut sketch "Sketch9" against normal blind 73.66 contours L358 L355 L356 L354 L353 L352
sketch "Sketch10" plane through (0, 0, 0) normal (0, -1, 0) x (1, 0, 0)
  line L0 (-8.861, 51.8104) -> (-8.861, 49.7896) projected
  line L1 (-5.4803, 49.7896) -> (-5.4803, 51.8104) projected
  line L2 (-7.1707, 52.8207) -> (-8.861, 51.8104) projected
  line L3 (-5.4803, 51.8104) -> (-7.1707, 52.8207) projected
  line L4 (-8.861, 49.7896) -> (-7.1707, 48.7793) projected
  line L5 (-7.1707, 48.7793) -> (-5.4803, 49.7896) projected
  line L6 (-8.3781, 26.1217) -> (-8.3781, 24.6783) projected
  line L7 (-7.1707, 26.8434) -> (-8.3781, 26.1217) projected
  line L8 (-5.9633, 26.1217) -> (-7.1707, 26.8434) projected
  line L9 (-5.9633, 24.6783) -> (-5.9633, 26.1217) projected
  line L10 (-7.1707, 23.9566) -> (-5.9633, 24.6783) projected
  line L11 (-8.3781, 24.6783) -> (-7.1707, 23.9566) projected
  line L12 (-8.1366, 0.5774) -> (-8.1366, -0.5774) projected
  line L13 (-6.2047, -0.5774) -> (-6.2047, 0.5774) projected
  line L14 (-6.2047, 0.5774) -> (-7.1707, 1.1547) projected
  line L15 (-7.1707, 1.1547) -> (-8.1366, 0.5774) projected
  line L16 (-8.1366, -0.5774) -> (-7.1707, -1.1547) projected
  line L17 (-7.1707, -1.1547) -> (-6.2047, -0.5774) projected
  line L18 (-8.3207, -24.7126) -> (-8.3207, -26.0874) projected
  line L19 (-7.1707, -24.0252) -> (-8.3207, -24.7126) projected
  line L20 (-6.0206, -24.7126) -> (-7.1707, -24.0252) projected
  line L21 (-6.0206, -26.0874) -> (-6.0206, -24.7126) projected
  line L22 (-8.3207, -26.0874) -> (-7.1707, -26.7748) projected
  line L23 (-7.1707, -26.7748) -> (-6.0206, -26.0874) projected
  line L24 (-7.9374, -50.3417) -> (-7.9374, -51.2583) projected
  line L25 (-7.1707, -49.8835) -> (-7.9374, -50.3417) projected
  line L26 (-6.404, -50.3417) -> (-7.1707, -49.8835) projected
  line L27 (-6.404, -51.2583) -> (-6.404, -50.3417) projected
  line L28 (-7.1707, -51.7165) -> (-6.404, -51.2583) projected
  line L29 (-7.9374, -51.2583) -> (-7.1707, -51.7165) projected
  line L30 (-28.5831, 49.7896) -> (-26.8927, 48.7793) projected
  line L31 (-28.5831, 51.8104) -> (-28.5831, 49.7896) projected
  line L32 (-26.8927, 52.8207) -> (-28.5831, 51.8104) projected
  line L33 (-25.2023, 51.8104) -> (-26.8927, 52.8207) projected
  line L34 (-25.2023, 49.7896) -> (-25.2023, 51.8104) projected
  line L35 (-26.8927, 48.7793) -> (-25.2023, 49.7896) projected
  line L36 (-28.1001, 24.6783) -> (-26.8927, 23.9566) projected
  line L37 (-28.1001, 26.1217) -> (-28.1001, 24.6783) projected
  line L38 (-26.8927, 26.8434) -> (-28.1001, 26.1217) projected
  line L39 (-25.6853, 26.1217) -> (-26.8927, 26.8434) projected
  line L40 (-25.6853, 24.6783) -> (-25.6853, 26.1217) projected
  line L41 (-26.8927, 23.9566) -> (-25.6853, 24.6783) projected
  line L42 (-27.8586, -0.5774) -> (-26.8927, -1.1547) projected
  line L43 (-27.8586, 0.5774) -> (-27.8586, -0.5774) projected
  line L44 (-26.8927, 1.1547) -> (-27.8586, 0.5774) projected
  line L45 (-25.9268, 0.5774) -> (-26.8927, 1.1547) projected
  line L46 (-25.9268, -0.5774) -> (-25.9268, 0.5774) projected
  line L47 (-26.8927, -1.1547) -> (-25.9268, -0.5774) projected
  line L48 (-28.0427, -26.0874) -> (-26.8927, -26.7748) projected
  line L49 (-28.0427, -24.7126) -> (-28.0427, -26.0874) projected
  line L50 (-26.8927, -24.0252) -> (-28.0427, -24.7126) projected
  line L51 (-25.7426, -24.7126) -> (-26.8927, -24.0252) projected
  line L52 (-25.7426, -26.0874) -> (-25.7426, -24.7126) projected
  line L53 (-26.8927, -26.7748) -> (-25.7426, -26.0874) projected
  line L54 (-26.126, -50.3417) -> (-26.8927, -49.8835) projected
  line L55 (-26.126, -51.2583) -> (-26.126, -50.3417) projected
  line L56 (-26.8927, -51.7165) -> (-26.126, -51.2583) projected
  line L57 (-27.6594, -51.2583) -> (-26.8927, -51.7165) projected
  line L58 (-27.6594, -50.3417) -> (-27.6594, -51.2583) projected
  line L59 (-26.8927, -49.8835) -> (-27.6594, -50.3417) projected
  arc A0 (-43.9323, 51.6673) -> (-45.7238, 48.8096) centre (-42.5488, 48.8096) ccw projected
  line L60 (-45.7238, -48.8096) -> (-45.7238, 48.8096) projected
  arc A1 (-45.7238, -48.8096) -> (-43.9323, -51.6673) centre (-42.5488, -48.8096) ccw projected
  line L61 (-2.3979, -71.7745) -> (-43.9323, -51.6673) projected
  arc A2 (-2.3979, -71.7745) -> (1.5596, -70.7755) centre (-1.0145, -68.9168) ccw projected
  line L62 (29.138, -32.5822) -> (1.5596, -70.7755) projected
  arc A3 (29.138, -32.5822) -> (29.7389, -30.7235) centre (26.5639, -30.7235) ccw projected
  line L63 (29.7389, 30.7235) -> (29.7389, -30.7235) projected
  arc A4 (29.7389, 30.7235) -> (29.138, 32.5822) centre (26.5639, 30.7235) ccw projected
  line L64 (1.5596, 70.7755) -> (29.138, 32.5822) projected
  arc A5 (1.5596, 70.7755) -> (-2.3979, 71.7745) centre (-1.0145, 68.9168) ccw projected
  line L65 (-43.9323, 51.6673) -> (-2.3979, 71.7745) projected
  line L66 (-1.6231, 66.5056) -> (24.6589, 30.1076) projected
  line L67 (24.6589, 30.1076) -> (24.6589, -30.1076) projected
  line L68 (24.6589, -30.1076) -> (-1.6231, -66.5056) projected
  line L69 (-1.6231, -66.5056) -> (-21.6786, -56.7965) projected
  line L70 (-21.6786, -56.7965) -> (-0.4003, -56.7965) projected
  line L71 (-0.4003, -56.7965) -> (-0.4003, 57.9007) projected
  line L72 (-0.4003, 57.9007) -> (-19.3978, 57.9007) projected
  line L73 (-19.3978, 57.9007) -> (-1.6231, 66.5056) projected
  line L74 (-0.4003, -56.7965) -> (-0.4003, 57.9007) projected
  line L75 (-40.6438, -44.8035) -> (-0.4003, -44.8035)
  line L76 (-0.4003, -44.8035) -> (-0.4003, -31.8548)
  line L77 (-0.4003, -31.8548) -> (-40.6438, -31.8548)
  line L78 (-40.6438, -31.8548) -> (-40.6438, -44.8035)
  line L79 (-40.6438, -18.9452) -> (-0.4003, -18.9452)
  line L80 (-0.4003, -18.9452) -> (-0.4003, -6.2347)
  line L81 (-0.4003, -6.2347) -> (-40.6438, -6.2347)
  line L82 (-40.6438, -6.2347) -> (-40.6438, -18.9452)
  line L83 (-40.6438, 6.2347) -> (-0.4003, 6.2347)
  line L84 (-0.4003, 6.2347) -> (-0.4003, 18.8766)
  line L85 (-0.4003, 18.8766) -> (-40.6438, 18.8766)
  line L86 (-40.6438, 18.8766) -> (-40.6438, 6.2347)
  line L87 (-40.6438, 31.9234) -> (-0.4003, 31.9234)
  line L88 (-0.4003, 31.9234) -> (-0.4003, 43.6993)
  line L89 (-0.4003, 43.6993) -> (-40.6438, 43.6993)
  line L90 (-40.6438, 43.6993) -> (-40.6438, 31.9234)
  line L91 (-0.4003, -56.7965) -> (-0.4003, 57.9007) projected
  point P0 (0, 0)
  dimension "d52" = 5.08
  dimension "d53" = 5.08
  dimension "d54" = 5.08
  dimension "d55" = 5.08
  dimension "d56" = 5.08
  dimension "d57" = 5.08
  dimension "d58" = 5.08
  dimension "d59" = 5.08
  dimension "d60" = 5.08
  constraints: 32 end point, 8 parallel, 6 point on line, 4 horizontal, 4 perpendicular, 1 collinear
  measures "d52" distance from line of L54.end L75
  measures "d53" distance from line of L48.end L77
  measures "d54" distance between parallel lines of L60 L78
  measures "d55" distance from line of L50.start L79
  measures "d56" distance from line of L42.end L81
  measures "d57" distance from line of L83 L44.start
  measures "d58" distance from line of L36.end L85
  measures "d59" distance from line of L87 L38.start
  measures "d60" distance from line of L30.end L89